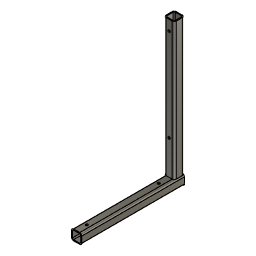
Podpěra - jekl v3 (Autodesk Fusion 360 design; units mm, degrees)
Autodesk Fusion 360 part; units mm, degrees
sketch "Sketch1" plane through (0, 0, 0) normal (0, 0, 1) x (1, 0, 0)
  line L0 (3, 15) -> (12, 15)
  line L1 (15, 12) -> (15, 3)
  line L2 (12, 0) -> (3, 0)
  line L3 (0, 3) -> (0, 12)
  arc A0 (3, 15) -> (0, 12) centre (3, 12) ccw
  arc A1 (15, 12) -> (12, 15) centre (12, 12) ccw
  arc A2 (12, 0) -> (15, 3) centre (12, 3) ccw
  arc A3 (0, 3) -> (3, 0) centre (3, 3) ccw
  line L4 (3, 13.5) -> (12, 13.5)
  arc A4 (13.5, 12) -> (12, 13.5) centre (12, 12) ccw
  line L5 (13.5, 12) -> (13.5, 3)
  arc A5 (12, 1.5) -> (13.5, 3) centre (12, 3) ccw
  line L6 (12, 1.5) -> (3, 1.5)
  arc A6 (1.5, 3) -> (3, 1.5) centre (3, 3) ccw
  line L7 (1.5, 3) -> (1.5, 12)
  arc A7 (3, 13.5) -> (1.5, 12) centre (3, 12) ccw
  point P0 (0, 15)
  point P1 (15, 15)
  point P2 (15, 0)
  dimension "d1" = 15
  dimension "d2" = 15
  dimension "d3" = 15
  dimension "d4" = 15
  dimension "d5" = 1.5
  dimension "d6" = 3
  constraint horizontal L0
  constraint vertical L1
  constraint horizontal L2
  constraint vertical L3
  constraint coincident P0 L0
  constraint coincident P0 L3
  constraint tangent L0 A0
  constraint tangent L3 A0
  constraint coincident P1 L0
  constraint coincident P1 L1
  constraint tangent L0 A1
  constraint tangent L1 A1
  constraint equal A0 A1
  constraint coincident P2 L1
  constraint coincident P2 L2
  constraint tangent L1 A2
  constraint tangent L2 A2
  constraint equal A0 A2
  constraint coincident origin L2
  constraint coincident origin L3
  constraint tangent L2 A3
  constraint tangent L3 A3
  constraint equal A0 A3
  measures "d1" vertical distance of origin P0
  measures "d2" distance of P0 origin
  measures "d3" distance of origin P2
  measures "d4" distance of P0 P1
  measures "d6" radius of A0
extrude "Extrude1" add sketch "Sketch1" along normal blind 200 makes body 1
sketch "Sketch2" plane through (0, 0, 0) normal (0, 1, 0) x (1, 0, 0)
  line L0 (3, -15) -> (12, -15)
  line L1 (15, -12) -> (15, -3)
  line L2 (12, 0) -> (3, 0)
  line L3 (0, -3) -> (0, -12)
  arc A0 (0, -12) -> (3, -15) centre (3, -12) ccw
  arc A1 (12, -15) -> (15, -12) centre (12, -12) ccw
  arc A2 (15, -3) -> (12, 0) centre (12, -3) ccw
  arc A3 (3, 0) -> (0, -3) centre (3, -3) ccw
  line L4 (3, -13.5) -> (12, -13.5)
  arc A4 (12, -13.5) -> (13.5, -12) centre (12, -12) ccw
  line L5 (13.5, -12) -> (13.5, -3)
  arc A5 (13.5, -3) -> (12, -1.5) centre (12, -3) ccw
  line L6 (12, -1.5) -> (3, -1.5)
  arc A6 (3, -1.5) -> (1.5, -3) centre (3, -3) ccw
  line L7 (1.5, -3) -> (1.5, -12)
  arc A7 (1.5, -12) -> (3, -13.5) centre (3, -12) ccw
  point P0 (0, -15)
  point P1 (15, -15)
  point P2 (15, 0)
  dimension "d9" = 15
  dimension "d10" = 15
  dimension "d11" = 15
  dimension "d12" = 15
  dimension "d13" = -1.5
  dimension "d14" = 3
  constraint horizontal L0
  constraint vertical L1
  constraint horizontal L2
  constraint vertical L3
  constraint coincident P0 L0
  constraint coincident P0 L3
  constraint tangent L0 A0
  constraint tangent L3 A0
  constraint coincident P1 L0
  constraint coincident P1 L1
  constraint tangent L0 A1
  constraint tangent L1 A1
  constraint equal A0 A1
  constraint coincident P2 L1
  constraint coincident P2 L2
  constraint tangent L1 A2
  constraint tangent L2 A2
  constraint equal A0 A2
  constraint tangent L2 A3
  constraint tangent L3 A3
  constraint equal A0 A3
  measures "d9" vertical distance of origin P0
  measures "d10" horizontal distance of origin P2
  measures "d11" distance of P0 P1
  measures "d12" distance of P1 P2
  measures "d14" radius of A0
extrude "Extrude2" add sketch "Sketch2" against normal blind 150 separate body makes body 2
move_body "Move1" bodies 1 to x (1, 0, 0) y (0, 1, 0) z (0, 0, 1) at (0, 0, 15)
move_body "Move2" bodies 2 to x (1, 0, 0) y (0, 1, 0) z (0, 0, 1) at (0, 15, 0)
sketch "Sketch3" plane through (0, 0, 15) normal (0, 0, 1) x (-1, 0, 0)
  line L0 (-12, -15) -> (-3, -15)
  line L1 (-3, -15) -> (-3, 135)
  line L2 (-3, 135) -> (-12, 135)
  line L3 (-12, 135) -> (-12, -15)
  circle A0 centre (-7.5, 15) radius 1.75
  circle A1 centre (-7.5, 120) radius 1.75
  line L4 (-15, -15) -> (-15, 135)
  point P0 (0, 135)
  dimension "d17" = 3.5
  dimension "d18" = 7.5
  dimension "d19" = 15
  dimension "d20" = 5
  dimension "d21" = 3.5
  dimension "d22" = 7.5
  dimension "d23" = 120
  dimension "d24" = 150
  dimension "d25" = 15
  measures "d17" diameter of A0
  measures "d18" horizontal distance of origin A0.centre
  measures "d19" vertical distance of origin A0.centre
  measures "d21" diameter of A1
  measures "d22" horizontal distance of origin A1.centre
  measures "d23" vertical distance of origin A1.centre
  measures "d24" distance of L4.start L4.end
  measures "d25" vertical distance of A1.centre L4.end
extrude "Extrude3" cut sketch "Sketch3" against normal blind 26 contours A0 | A1 bodies 2
sketch "Sketch4" plane through (0, 0, 0) normal (0, -1, 0) x (1, 0, 0)
  line L0 (3, 15) -> (12, 15)
  line L1 (12, 15) -> (12, 215)
  line L2 (12, 215) -> (3, 215)
  line L3 (3, 215) -> (3, 15)
  circle A0 centre (7.5, 200) radius 1.75
  circle A1 centre (7.5, 65) radius 1.75
  dimension "d28" = 3.5
  dimension "d29" = 15
  dimension "d30" = 7.5
  dimension "d31" = 3.5
  dimension "d32" = 7.5
  dimension "d33" = 135
  measures "d28" diameter of A0
  measures "d29" distance of L2 A0.centre
  measures "d30" horizontal distance of origin A0.centre
  measures "d31" diameter of A1
  measures "d32" horizontal distance of origin A1.centre
  measures "d33" distance of A0.centre A1.centre
extrude "Extrude4" cut sketch "Sketch4" against normal blind 35 contours A0 | A1 bodies 1
